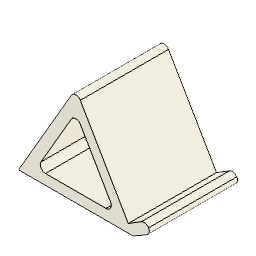
top11 (Autodesk Fusion 360 design; units mm, degrees)
part number: 2025-10-01-13-58-44-558
Autodesk Fusion 360 part; units mm, degrees
sketch "Sketch1" plane through (0, 0, 0) normal (0, 0, 1) x (1, 0, 0)
  line L0 (5, 0) -> (306, 0)
  line L1 (311, 5) -> (311, 200)
  line L2 (306, 205) -> (5, 205)
  line L3 (0, 200) -> (0, 5)
  arc A0 (5, 205) -> (0, 200) centre (5, 200) ccw
  arc A1 (311, 200) -> (306, 205) centre (306, 200) ccw
  arc A2 (0, 5) -> (5, 0) centre (5, 5) ccw
  arc A3 (306, 0) -> (311, 5) centre (306, 5) ccw
  line L4 (5, 0) -> (306, 0)
  line L5 (311, 5) -> (311, 56.5)
  line L6 (311, 56.5) -> (0, 56.5)
  line L7 (0, 56.5) -> (0, 5)
  arc A4 (0, 5) -> (5, 0) centre (5, 5) ccw
  arc A5 (306, 0) -> (311, 5) centre (306, 5) ccw
  line L8 (0, 148.5) -> (311, 148.5)
  line L9 (311, 148.5) -> (311, 200)
  line L10 (306, 205) -> (5, 205)
  line L11 (0, 200) -> (0, 148.5)
  arc A6 (5, 205) -> (0, 200) centre (5, 200) ccw
  arc A7 (311, 200) -> (306, 205) centre (306, 200) ccw
  point P0 (311, 0)
  point P1 (311, 0)
  dimension "d1" = 311
  dimension "d2" = 205
  dimension "d3" = 5
  dimension "d4" = 5
  dimension "d5" = 5
  dimension "d6" = 5
  dimension "d7" = 311
  dimension "d8" = 5
  dimension "d9" = 5
  dimension "d10" = 311
  dimension "d11" = 5
  dimension "d12" = 5
  dimension "d13" = 56.5
  dimension "d14" = 56.5
  constraint horizontal L0
  constraint vertical L1
  constraint horizontal L2
  constraint vertical L3
  constraint tangent L2 A0
  constraint tangent L3 A0
  constraint tangent L1 A1
  constraint tangent L2 A1
  constraint coincident origin L0
  constraint coincident origin L3
  constraint tangent L0 A2
  constraint tangent L3 A2
  constraint coincident P1 L0
  constraint coincident P1 L1
  constraint tangent L0 A3
  constraint tangent L1 A3
  constraint horizontal L4
  constraint vertical L5
  constraint horizontal L6
  constraint vertical L7
  constraint coincident origin L4
  constraint coincident origin L7
  constraint tangent L4 A4
  constraint tangent L7 A4
  constraint coincident P1 L4
  constraint coincident P1 L5
  constraint tangent L4 A5
  constraint tangent L5 A5
  constraint horizontal L8
  constraint vertical L9
  constraint horizontal L10
  constraint vertical L11
  constraint coincident L3 L8.start
  constraint tangent L10 A6
  constraint tangent L11 A6
  constraint tangent L9 A7
  constraint tangent L10 A7
  measures "d1" distance of origin P0
  measures "d2" distance of L0 L2
  measures "d3" radius of A0
  measures "d4" radius of A1
  measures "d5" radius of A2
  measures "d6" radius of A3
  measures "d7" distance of origin P1
  measures "d8" radius of A4
  measures "d9" radius of A5
  measures "d10" distance of L8.start L8.end
  measures "d11" radius of A6
  measures "d12" radius of A7
  measures "d13" distance of L8 L10
  measures "d14" distance of L4 L6
sketch "Sketch2" plane through (0, 0, 0) normal (0, 1, 0) x (1, 0, 0)
  line L0 (0, 0) -> (50.8661, -87.6955)
  line L1 (59.5163, -87.6955) -> (110.3824, 0)
  line L2 (110.3824, 0) -> (0, 0)
  line L3 (21.716, -17.5087) -> (50.8661, -67.7648)
  line L4 (59.5163, -67.7648) -> (88.6664, -17.5087)
  line L5 (84.3413, -10) -> (26.0411, -10)
  arc A0 (50.8661, -87.6955) -> (59.5163, -87.6955) centre (55.1912, -85.1868) ccw
  arc A1 (50.8661, -67.7648) -> (59.5163, -67.7648) centre (55.1912, -65.2561) ccw
  line L6 (110.3824, 0) -> (123.3577, -7.5261)
  line L7 (125.1741, -14.3599) -> (125.2504, -14.2282)
  arc A2 (125.1741, -14.3599) -> (123.3577, -7.5261) centre (120.849, -11.8512) ccw
  line L8 (105.6659, -8.1314) -> (118.2881, -15.9675)
  arc A3 (118.2881, -15.9675) -> (125.2504, -14.2282) centre (120.9253, -11.7195) ccw
  arc A4 (26.0411, -10) -> (21.716, -17.5087) centre (26.0411, -15) ccw
  arc A5 (88.6664, -17.5087) -> (84.3413, -10) centre (84.3413, -15) ccw
  point P0 (55.1912, -95.1522)
  point P1 (127.6828, -10.0348)
  point P2 (122.6654, -18.685)
  dimension "d15" = 110
  dimension "d16" = 110
  dimension "d18" = 5
  dimension "d19" = 5
  dimension "d20" = 20
  dimension "d21" = 10
  dimension "d22" = 5
  dimension "d23" = 5
  dimension "d24" = 5
  dimension "d25" = 5
  constraint coincident L0.start L2.end
  constraint horizontal L2
  constraint coincident P0 L0
  constraint coincident P0 L1
  constraint tangent L0 A0
  constraint tangent L1 A0
  constraint tangent L3 A1
  constraint tangent L4 A1
  constraint perpendicular L1 L6
  constraint perpendicular L6 L7
  constraint coincident P1 L6
  constraint coincident P1 L7
  constraint tangent L6 A2
  constraint tangent L7 A2
  constraint coincident L1 L8.start
  constraint coincident P2 L7
  constraint coincident P2 L8
  constraint tangent L7 A3
  constraint tangent L8 A3
  constraint tangent L3 A4
  constraint tangent L5 A4
  constraint tangent L4 A5
  constraint tangent L5 A5
  measures "d15" distance of L0.start P0
  measures "d16" distance of P0 L1.end
  measures "d18" radius of A0
  measures "d19" radius of A1
  measures "d20" distance of L1.end P1
  measures "d21" distance of P1 P2
  measures "d22" radius of A2
  measures "d23" radius of A3
  measures "d24" radius of A4
  measures "d25" radius of A5
form "Form1" [no effect]
extrude "Extrude1" add sketch "Sketch2" along normal blind 85
sketch "Sketch3" plane through (0, 0, 10) normal (0, 0, 1) x (-1, 0, 0)
  line L0 (-26.0411, 0) -> (-84.3413, 0)
  line L1 (-84.3413, 0) -> (-84.3413, -85)
  line L2 (-84.3413, -85) -> (-26.0411, -85)
  line L3 (-26.0411, -85) -> (-26.0411, 0)
